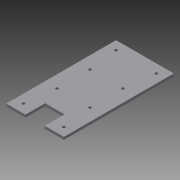
# Autodesk Inventor part: TopBase
Saved by Autodesk Inventor 2015 (Build 190159000, 159)
## iProperties
Created: 2015-04-04
Part Number: TopBase
Material: Generic
Document SubType Name: Modeling
Designer: Judson
Density: 1 g/cm^3
Appearance: Default
Author: Judson
Autodesk Inventor part; units mm, degrees
ref_plane "YZ Plane" through (0, 0, 0) normal (1, 0, 0) x (0, 1, 0)
ref_plane "XZ Plane" through (0, 0, 0) normal (0, 1, 0) x (-1, 0, 0)
ref_plane "XY Plane" through (0, 0, 0) normal (0, 0, 1) x (1, 0, 0)
sketch "Sketch1" plane through (0, 0, 0) normal (0, 1, 0) x (-1, 0, 0)
  line L0 (66.675, 127) -> (-66.675, 127)
  line L1 (-66.675, 127) -> (-66.675, -127)
  line L2 (-66.675, -127) -> (66.675, -127)
  line L3 (66.675, -127) -> (66.675, 127)
  point P0 (0, 0)
  dimension "d0" = 66.675
  dimension "d1" = 133.35
  dimension "d2" = 254
  dimension "d3" = 127
  constraints: 8 end point, 2 parallel, 1 horizontal, 1 perpendicular
  measures "d0" distance from line of point (0, 0) L3
  measures "d1" distance of L0.start L0.end
  measures "d2" distance of L2.end L0.start
  measures "d3" distance from line of point (0, 0) L0
extrude "Extrusion1" add sketch "Sketch1" along normal blind 5.9944
sketch "Sketch2" plane through (0, 5.9944, 0) normal (0, 1, 0) x (1, 0, 0)
  line L0 (-66.675, -127) -> (-66.675, 127) projected
  line L1 (-66.675, 127) -> (66.675, 127) projected
  line L2 (66.675, 127) -> (66.675, -127) projected
  line L3 (66.675, -127) -> (-66.675, -127) projected
  circle A0 centre (-46.675, -107) radius 3.175
  line L4 (-66.675, -127) -> (66.675, -127) projected
  line L5 (0, -127) -> (0, 127)
  line L6 (-66.675, 0) -> (66.675, 0)
  circle A1 centre (-46.675, 107) radius 3.175
  circle A2 centre (46.675, -107) radius 3.175
  circle A3 centre (46.675, 107) radius 3.175
  point P0 (0, 0)
  dimension "d6" = 20
  dimension "d7" = 20
  dimension "d8" = 6.35
  constraints: 4 centre point, 4 end point, 4 midpoint, 3 symmetric about line, 3 other
  measures "d6" distance from line of L0 A0.centre
  measures "d7" distance from line of L3 A0.centre
  measures "d8" diameter of A0
extrude "Extrusion2" cut sketch "Sketch2" against normal blind 5.9944 contours A0 | A1 | A2 | A3
sketch "Sketch3" plane through (0, 5.9944, 0) normal (0, 1, 0) x (1, 0, 0)
  circle A0 centre (-46.675, -107) radius 3.175 projected
  circle A1 centre (46.675, -107) radius 3.175 projected
  circle A2 centre (46.675, 107) radius 3.175 projected
  circle A3 centre (-46.675, 107) radius 3.175 projected
  line L0 (-66.675, -127) -> (-66.675, 127) projected
  line L1 (-66.675, 127) -> (66.675, 127) projected
  line L2 (66.675, 127) -> (66.675, -127) projected
  line L3 (66.675, -127) -> (-66.675, -127) projected
  line L4 (-66.675, 0) -> (66.675, 0)
  line L5 (66.675, 127) -> (-66.675, 127) projected
  line L6 (0, 127) -> (0, -127)
  line L7 (-66.675, -127) -> (66.675, -127) projected
  circle A4 centre (-38.1, -38.1) radius 3.175
  circle A5 centre (-38.1, 38.1) radius 3.175
  circle A6 centre (38.1, -38.1) radius 3.175
  circle A7 centre (38.1, 38.1) radius 3.175
  point P0 (0, 0)
  dimension "d11" = 6.35
  dimension "d12" = 38.1
  dimension "d13" = 38.1
  constraints: 4 centre point, 4 end point, 4 midpoint, 3 symmetric about line, 3 other
  measures "d11" diameter of A4
  measures "d12" distance from line of L4 A4.centre
  measures "d13" distance from line of L6 A4.centre
extrude "Extrusion3" cut sketch "Sketch3" against normal blind 5.9944 contours A4 | A5 | A6 | A7
sketch "Sketch4" plane through (0, 5.9944, 0) normal (0, 1, 0) x (1, 0, 0)
  circle A0 centre (-38.1, 38.1) radius 3.175 projected
  circle A1 centre (38.1, -38.1) radius 3.175 projected
  circle A2 centre (38.1, 38.1) radius 3.175 projected
  circle A3 centre (-38.1, -38.1) radius 3.175 projected
  circle A4 centre (-46.675, -107) radius 3.175 projected
  circle A5 centre (46.675, -107) radius 3.175 projected
  circle A6 centre (46.675, 107) radius 3.175 projected
  circle A7 centre (-46.675, 107) radius 3.175 projected
  line L0 (-66.675, -127) -> (-66.675, 127) projected
  line L1 (-66.675, 127) -> (66.675, 127) projected
  line L2 (66.675, 127) -> (66.675, -127) projected
  line L3 (66.675, -127) -> (-66.675, -127) projected
  line L4 (-22.225, -127) -> (22.225, -127)
  line L5 (22.225, -127) -> (22.225, -81.28)
  line L6 (22.225, -81.28) -> (-22.225, -81.28)
  line L7 (-22.225, -81.28) -> (-22.225, -127)
  line L8 (0, -127) -> (0, 0)
  dimension "d16" = 22.225
  dimension "d17" = 22.225
  dimension "d18" = 45.72
  constraints: 10 end point, 2 parallel, 2 perpendicular, 1 horizontal, 1 midpoint, 1 point on line
  measures "d16" distance between parallel lines of L7 L8
  measures "d17" distance between parallel lines of L5 L8
  measures "d18" distance between parallel lines of L3 L6
extrude "Extrusion4" cut sketch "Sketch4" against normal blind 5.9944 contours L7 L6 L8 L3 | L8 L6 L5 L3
body "Solid1"
